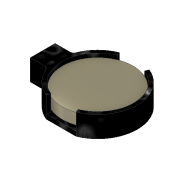
# Autodesk Inventor part: Keystone_1070
Saved by Autodesk Inventor 2017 (Build 210142000, 142)
## iProperties
Part Number: Keystone_1070
Material: Generisch
Document SubType Name: Modeling
Designer: David Merges
Density: 1 g/cm^3
Appearance: Schwarz
Author: David Merges
Autodesk Inventor part; units mm, degrees
ref_plane "YZ Plane" through (0, 0, 0) normal (1, 0, 0) x (0, 1, 0)
ref_plane "XZ Plane" through (0, 0, 0) normal (0, 1, 0) x (-1, 0, 0)
sketch "Skizze1" plane through (0, 0, 0) normal (0, 0, 1) x (1, 0, 0)
  line L0 (-4.214, 10.35) -> (4.214, 10.35)
  line L1 (-4.214, -10.35) -> (4.214, -10.35)
  line L2 (-11.3129, 3.5) -> (-15.55, 3.5)
  line L3 (-15.55, 3.5) -> (-15.55, -3.5)
  line L4 (-15.55, -3.5) -> (-11.3129, -3.5)
  arc A0 (-10.3837, -4.1304) -> (-4.214, -10.35) centre (0, 0) ccw
  arc A1 (-4.214, 10.35) -> (-10.3837, 4.1304) centre (0, 0) ccw
  arc A2 (4.214, -10.35) -> (4.214, 10.35) centre (0, 0) ccw
  line L5 (-15.55, 0) -> (0, 0) construction
  arc A3 (-11.3129, 3.5) -> (-10.3837, 4.1304) centre (-11.3129, 4.5) ccw
  arc A4 (-10.3837, -4.1304) -> (-11.3129, -3.5) centre (-11.3129, -4.5) ccw
  point P0 (-10.6128, -3.5)
  point P1 (-10.6128, 3.5)
  dimension "d0" = 7
  dimension "d1" = 20.7
  dimension "d2" = 11.175
  dimension "d5" = 1
  dimension "d6" = 15.55
  constraints: 12 end point, 12 point on circle, 5 centre point, 4 horizontal, 4 tangent, 3 coincident, 3 equal radius, 2 parallel, 2 perpendicular, 2 point on line, 1 midpoint
  measures "d0" distance between parallel lines of L2 L4
  measures "d1" distance between parallel lines of L0 L1
  measures "d2" radius of A0
  measures "d5" radius of A3
  measures "d6" distance from line of L3 L5.end
extrude "Extrusion1" add sketch "Skizze1" along normal blind 1.27
sketch "Skizze2" plane through (0, 0, 1.27) normal (0, 0, 1) x (1, 0, 0)
  line L0 (4.214, 10.35) -> (-4.214, 10.35) projected
  arc A0 (-4.214, 10.35) -> (-10.3837, 4.1304) centre (0, 0) ccw projected
  arc A1 (-11.3129, 3.5) -> (-10.3837, 4.1304) centre (-11.3129, 4.5) ccw projected
  line L1 (-11.3129, 3.5) -> (-15.55, 3.5) projected
  line L2 (-15.55, 3.5) -> (-15.55, -3.5) projected
  line L3 (-15.55, -3.5) -> (-11.3129, -3.5) projected
  arc A2 (-10.3837, -4.1304) -> (-11.3129, -3.5) centre (-11.3129, -4.5) ccw projected
  arc A3 (-10.3837, -4.1304) -> (-4.214, -10.35) centre (0, 0) ccw projected
  line L4 (-4.214, -10.35) -> (4.214, -10.35) projected
  arc A4 (4.214, -10.35) -> (4.214, 10.35) centre (0, 0) ccw projected
  arc A5 (-3.8219, 9.3868) -> (-3.8219, -9.3868) centre (0, 0) ccw
  arc A6 (3.8219, -9.3868) -> (3.8219, 9.3868) centre (0, 0) ccw
  line L5 (-4.214, 10.35) -> (-3.8219, 9.3868)
  line L6 (3.8219, 9.3868) -> (4.214, 10.35)
  line L7 (-4.214, -10.35) -> (-3.8219, -9.3868)
  line L8 (4.214, -10.35) -> (3.8219, -9.3868)
  dimension "d7" = 10.135
  constraints: 8 end point, 4 point on circle, 4 point on line, 3 coincident, 2 centre point, 1 concentric
  measures "d7" radius of A5
extrude "Extrusion2" add sketch "Skizze2" along normal blind 4.7 contours A4 L8 A6 L6 | L5 A5 L7 A3 A2 L3 L2 L1 A1 A0
ref_plane "Arbeitsebene1" through (0, 0, 4.97) normal (0, 0, 1) x (1, 0, 0)
sketch "Skizze3" plane through (0, 0, 4.97) normal (0, 0, 1) x (1, 0, 0)
  circle A0 centre (0, 0) radius 10
  dimension "d11" = 20
  constraints: 1 centre point, 1 coincident
  measures "d11" diameter of A0
extrude "Extrusion3" add sketch "Skizze3" against normal blind 3.1
